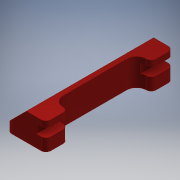
# Autodesk Inventor part: Payload_CameraSupport
Saved by Autodesk Inventor 2018 (Build 220112000, 112)
## iProperties
Created: 2018-07-29
Part Number: Payload_CameraSupport
Material: Aluminum
Document SubType Name: Modeling
Designer: Bradley
Density: 2.7 g/cm^3
Appearance: Anodized - Red
Author: Bradley
Autodesk Inventor part; units mm, degrees
ref_plane "YZ Plane" through (0, 0, 0) normal (1, 0, 0) x (0, 1, 0)
ref_plane "XZ Plane" through (0, 0, 0) normal (0, 1, 0) x (-1, 0, 0)
ref_plane "XY Plane" through (0, 0, 0) normal (0, 0, 1) x (1, 0, 0)
sketch "Sketch1" plane through (0, 0, 0) normal (0, 0, 1) x (1, 0, 0)
  line L0 (-4, 13) -> (-4, -13)
  line L1 (-4, -13) -> (4, -13)
  line L2 (4, -13) -> (4, 13)
  line L3 (4, 13) -> (-4, 13)
  line L4 (-1, -10) -> (-1, 10) construction
  circle A0 centre (-1, 10) radius 3 construction
  point P0 (0, 0)
  point P1 (0, 13)
  point P2 (-4, 0)
  point P3 (-1, 0)
  dimension "d0" = 26
  dimension "d2" = 20
  dimension "d5" = 5
  constraints: 10 end point, 3 midpoint, 2 horizontal alignment, 2 perpendicular, 2 tangent, 2 vertical, 1 centre point, 1 coincident, 1 horizontal, 1 vertical alignment
  measures "d0" distance of L0.start L0.end
  measures "d2" distance of L4.start L4.end
  measures "d5" distance from line of L2 L4.end
extrude "Extrusion1" add sketch "Sketch1" along normal mid plane 5.5
sketch "Sketch2" plane through (0, 0, 2.75) normal (0, 0, 1) x (1, 0, 0)
  point P0 (0, 0)
  point P1 (-1, 10)
  point P2 (-1, -10)
hole "Hole1" at (-1, 10, 2.75) at (-1, -10, 2.75) direction (0, 0, -1) diameter 1.567 end through all thread size "M2x0.4" class "6H" standard "ANSI Metric M Profile"
sketch "Sketch3" plane through (-4, -13, 2.75) normal (0, -1, 0) x (1, 0, 0)
  line L0 (8, -5.5) -> (8, 0) projected
  line L1 (0, 0) -> (8, 0) projected
  line L2 (0, -5.5) -> (0, 0) projected
  line L3 (8, -5.5) -> (0, -5.5) projected
  line L4 (8, -5.5) -> (8, 0) projected
  line L5 (8, -1.2) -> (6, -1.2)
  line L6 (6, -1.2) -> (6, -3)
  line L7 (6, -3) -> (8, -3)
  line L8 (8, -3) -> (8, -1.2)
  point P0 (4, -2.75)
  dimension "d13" = 2.5
  dimension "d14" = 1.8
  dimension "d15" = 2
  constraints: 8 end point, 2 parallel, 1 horizontal, 1 perpendicular, 1 point on line
  measures "d13" distance between parallel lines of L3 L7
  measures "d14" distance of L5.end L6.end
  measures "d15" distance of L5.start L5.end
extrude "Extrusion2" cut sketch "Sketch3" against normal through all contours L7 L6 L5 L0
chamfer "Chamfer1" distance 4 angle 45 1 edges at (-4, 0, 2.75)
sketch "Sketch4" plane through (0, 0, 2.75) normal (0, 0, 1) x (1, 0, 0)
  line L0 (0, -13) -> (0, 13) projected
  line L1 (0, -13) -> (4, -13) projected
  line L2 (4, -13) -> (4, 13) projected
  line L3 (4, 13) -> (0, 13) projected
  line L4 (4, 13) -> (4, -13) projected
  line L5 (4, 8.5) -> (1, 8.5)
  line L6 (1, 8.5) -> (1, -8.5)
  line L7 (1, -8.5) -> (4, -8.5)
  line L8 (4, -8.5) -> (4, 8.5)
  line L9 (4, -13) -> (4, 13) projected
  point P0 (0, 0)
  point P1 (4, 0)
  dimension "d21" = 3
  dimension "d22" = 17
  constraints: 8 end point, 2 midpoint, 2 parallel, 1 horizontal, 1 perpendicular, 1 point on line
  measures "d21" distance of L7.end L6.end
  measures "d22" distance of L6.end L5.end
extrude "Extrusion3" cut sketch "Sketch4" against normal through all contours L7 L6 L5 L2
fillet "Fillet1" radius 2 2 edges at (1, 8.5, 0) (1, -8.5, 0)
fillet "Fillet1" radius 1 10 edges at (4, -8.5, 2.15) (4, -13, 2.15) (4, -13, -1.5) (4, -8.5, -1.5) (4, 13, 2.15) (4, 8.5, 2.15) (4, 8.5, -1.5) (4, 13, -1.5) (-4, 13, -2) (-4, -13, -2)
body "Solid1"
